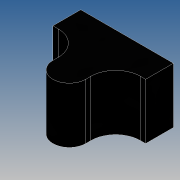
# Autodesk Inventor part: Boton de temperaturas
Saved by Autodesk Inventor 2016 (Build 200138000, 138)
## iProperties
Created: 2016-05-25
Part Number: Boton de temperaturas
Material: ABS Plastic
Document SubType Name: Modeling
Designer: Familia
Density: 1.06 g/cm^3
Appearance: Black
Mass: 0.59444 g
Surface Area: 12.396 cm^2
Volume: 0.560793 cm^3
Author: Familia
Autodesk Inventor part; units mm, degrees
ref_plane "YZ Plane" through (0, 0, 0) normal (1, 0, 0) x (0, 1, 0)
ref_plane "XZ Plane" through (0, 0, 0) normal (0, 1, 0) x (-1, 0, 0)
ref_plane "XY Plane" through (0, 0, 0) normal (0, 0, 1) x (1, 0, 0)
sketch "Sketch1" plane through (0, 0, 0) normal (0, 0, 1) x (1, 0, 0)
  arc A0 (-2.65, 0) -> (2.65, 0) centre (0, 0) ccw
  line L0 (-7.5, 9.35) -> (7.5, 9.35)
  line L1 (7.5, 9.35) -> (7.5, 4.85)
  line L2 (-7.5, 4.85) -> (-7.5, 9.35)
  line L3 (-2.65, 0) -> (-2.65, 0.85)
  line L4 (2.65, 0.85) -> (2.65, 0)
  line L5 (7.5, 4.85) -> (6.65, 4.85)
  line L6 (-6.65, 4.85) -> (-7.5, 4.85)
  line L7 (0, 0) -> (0, 9.35) construction
  arc A1 (-2.65, 0.85) -> (-6.65, 4.85) centre (-6.65, 0.85) ccw
  arc A2 (6.65, 4.85) -> (2.65, 0.85) centre (6.65, 0.85) ccw
  dimension "d0" = 2.65
  dimension "d1" = 4.5
  dimension "d2" = 15
  dimension "d3" = 12
  dimension "d4" = 4
  constraints: 16 end point, 6 point on circle, 6 tangent, 3 centre point, 3 parallel, 3 vertical, 1 coincident, 1 collinear, 1 equal radius, 1 horizontal, 1 midpoint, 1 perpendicular
  measures "d0" radius of A0
  measures "d1" distance of L2.start L0.start
  measures "d2" distance of L0.start L0.end
  measures "d4" radius of A1
extrude "Extrusion1" add sketch "Sketch1" along normal blind 9
shell "Shell1" thickness 1 removed faces 1 at (-2.5, 9.35, 3)
sketch "Sketch3" plane through (-7.5, 9.35, 0) normal (0, 1, 0) x (1, 0, 0)
  line L0 (1, -5.1) -> (1, -3.9)
  line L1 (14, -3.9) -> (14, -5.1)
  line L2 (11, -2.1) -> (4, -2.1)
  line L3 (4, -6.9) -> (11, -6.9)
  line L4 (11, -2.1) -> (4, -6.9) construction
  line L5 (4, -2.1) -> (11, -6.9) construction
  line L6 (14, -5.1) -> (11, -5.1)
  line L7 (4, -5.1) -> (1, -5.1)
  line L8 (1, -3.9) -> (4, -3.9)
  line L9 (11, -3.9) -> (14, -3.9)
  line L10 (4, -2.1) -> (4, -3.9)
  line L11 (4, -5.1) -> (4, -6.9)
  line L12 (11, -6.9) -> (11, -5.1)
  line L13 (11, -3.9) -> (11, -2.1)
  line L14 (14, -1) -> (14, -8) projected
  line L15 (1, -8) -> (1, -1) projected
  line L16 (14, -8) -> (1, -8) projected
  line L17 (7.5, -8) -> (7.5, -4.5) construction
  line L18 (1, -1) -> (14, -1) projected
  line L19 (7.5, -1) -> (7.5, -4.5) construction
  line L20 (4.8, -2.6486) -> (10.2, -2.6486)
  line L21 (10.2, -2.6486) -> (10.2, -6.3514)
  line L22 (10.2, -6.3514) -> (4.8, -6.3514)
  line L23 (4.8, -6.3514) -> (4.8, -2.6486)
  line L24 (4.8, -2.6486) -> (10.2, -6.3514) construction
  line L25 (10.2, -2.6486) -> (4.8, -6.3514) construction
  point P0 (7.5, 0)
  dimension "d8" = 1.2
  dimension "d9" = 7
  dimension "d10" = 4.8
  dimension "d11" = 0.8
  constraints: 44 end point, 12 parallel, 8 collinear, 8 midpoint, 5 perpendicular, 4 horizontal, 1 point on line, 1 vertical
  measures "d8" distance of L1.start L1.end
  measures "d9" distance of L3.start L3.end
  measures "d10" distance between parallel lines of L2 L3
  measures "d11" distance between parallel lines of L21 L12
extrude "Extrusion2" add sketch "Sketch3" against normal up to next contours L0 L8 L10 L2 L13 L9 L1 L6 L12 L3 L11 L7
body "Solid1"
